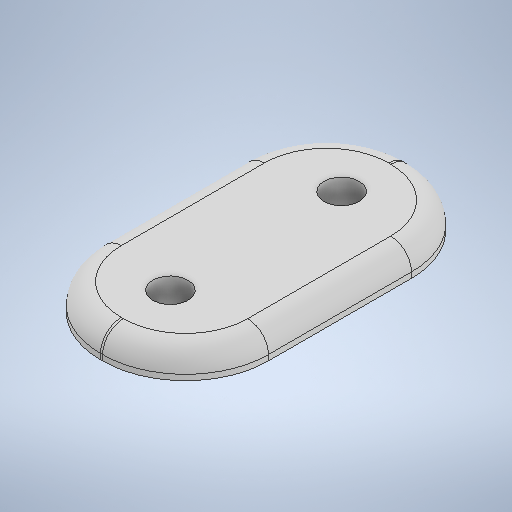
# Autodesk Inventor part: Part1
Saved by Autodesk Inventor 2025.3 (Build 293356000, 356)
## iProperties
Created: 2025-07-14
Part Number: Part1
Material: Generic
Document SubType Name: Modeling
Designer: steve
Density: 1 g/cm^3
Appearance: Default
Author: steve
Autodesk Inventor part; units mm, degrees
ref_plane "YZ Plane" through (0, 0, 0) normal (1, 0, 0) x (0, 1, 0)
ref_plane "XZ Plane" through (0, 0, 0) normal (0, 1, 0) x (-1, 0, 0)
ref_plane "XY Plane" through (0, 0, 0) normal (0, 0, 1) x (1, 0, 0)
sketch "Sketch1" plane through (0, 0, 0) normal (0, 1, 0) x (-1, 0, 0)
  circle A0 centre (0, 0) radius 1.27
  line L0 (0, 1.27) -> (0, 4.98) construction
  line L1 (0, 4.98) -> (0, -17.37) construction
  line L2 (0, -6.195) -> (6.075, -6.195) construction
  line L3 (0, 4.98) -> (0.075, 4.98)
  line L4 (6.075, -1.02) -> (6.075, -6.195)
  line L5 (0, 4.98) -> (-0.075, 4.98)
  line L6 (-6.075, -1.02) -> (-6.075, -6.195)
  line L7 (-6.075, -6.195) -> (0, -6.195) construction
  arc A1 (6.075, -1.02) -> (0.075, 4.98) centre (0.075, -1.02) ccw
  arc A2 (-0.075, 4.98) -> (-6.075, -1.02) centre (-0.075, -1.02) ccw
  circle A3 centre (0, -12.39) radius 1.27
  line L8 (0, -13.66) -> (0, -17.37) construction
  line L9 (0, -17.37) -> (0, 4.98) construction
  line L10 (0, -17.37) -> (0.075, -17.37)
  line L11 (0, -17.37) -> (-0.075, -17.37)
  arc A4 (0.075, -17.37) -> (6.075, -11.37) centre (0.075, -11.37) ccw
  arc A5 (-6.075, -11.37) -> (-0.075, -17.37) centre (-0.075, -11.37) ccw
  line L12 (6.075, -11.37) -> (6.075, -6.195)
  line L13 (-6.075, -11.37) -> (-6.075, -6.195)
  point P0 (-6.075, 4.98)
  point P1 (-6.075, -17.37)
  point P2 (6.075, -3.6075)
  dimension "d0" = 2.54
  dimension "d1" = 3.71
  dimension "d2" = 22.35
  dimension "d3" = 6.075
  dimension "d4" = 6.075
  dimension "d5" = 6
  dimension "d6" = 6
  dimension "d7" = 12.15
  constraints: 28 end point, 12 symmetric about line, 8 point on circle, 5 point on line, 4 centre point, 4 tangent, 3 horizontal, 3 perpendicular, 3 vertical, 2 coincident, 2 midpoint, 2 vertical alignment, 1 parallel, 6 other
  measures "d1" distance of L0.start L0.end
  measures "d2" distance of L0.end L1.end
  measures "d3" distance of L2.start L2.end
  measures "d4" distance of L0.end point (-6.075, 4.98)
  measures "d5" radius of A1
  measures "d6" radius of A2
  measures "d7" distance from line of L6 point (6.075, -3.608)
extrude "Extrusion1" add sketch "Sketch1" along normal blind 1.9
fillet "Fillet1" radius 1.5 8 edges at (6.075, 1.9, -3.6075) (4.3176, 1.9, -15.6126) (-0.0375, 1.9, -17.37) (-4.3176, 1.9, -15.6126) (-6.075, 1.9, -3.6075) (-4.3176, 1.9, 3.2226) (-0.0375, 1.9, 4.98) (4.3176, 1.9, 3.2226)
body "Solid1"
